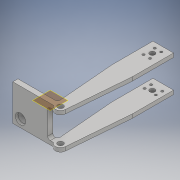
# Autodesk Inventor part: WheelIntakeMount3.0
Saved by Autodesk Inventor 2017 (Build 210142000, 142)
## iProperties
Created: 2017-12-06
Part Number: WheelIntakeMount3.0
Material: Generic
Document SubType Name: Modeling
Designer: User
Density: 1 g/cm^3
Appearance: Default
Author: User
Autodesk Inventor part; units mm, degrees
ref_plane "YZ Plane" through (0, 0, 0) normal (1, 0, 0) x (0, 1, 0)
ref_plane "XZ Plane" through (0, 0, 0) normal (0, 1, 0) x (-1, 0, 0)
ref_plane "XY Plane" through (0, 0, 0) normal (0, 0, 1) x (1, 0, 0)
sketch "Sketch1" plane through (0, 0, 0) normal (1, 0, 0) x (0, 1, 0)
  line L0 (0, 0) -> (127, 0)
  line L1 (127, 0) -> (127, -25.4)
  line L2 (127, -25.4) -> (0, -25.4)
  line L3 (0, -25.4) -> (0, 0)
  line L4 (0, -6.35) -> (0, -19.05)
  line L5 (0, -6.35) -> (76.2, 0)
  line L6 (0, -19.05) -> (76.2, -25.4)
  dimension "d0" = 127
  dimension "d1" = 25.4
  dimension "d18" = 12.7
  dimension "d19" = 6.35
  dimension "d20" = 50.8
  dimension "d21" = 50.8
  constraints: 14 end point, 4 point on line, 2 parallel, 1 horizontal, 1 perpendicular
  measures "d0" distance of L1.end L2.end
  measures "d1" distance of L0.end L1.end
  measures "d18" distance of L4.start L4.end
  measures "d19" distance from line of L2 L4.end
  measures "d20" distance from line of L1 L6.end
  measures "d21" distance from line of L5.end L1
ref_plane "Work Plane1" through (44.5262, 0, 0) normal (1, 0, 0) x (0, 0, -1)
sketch "Sketch2" plane through (44.5262, 0, 0) normal (1, 0, 0) x (0, 0, -1)
  line L0 (0, 127) -> (0, 0) projected
  line L1 (0, 0) -> (25.4, 0) projected
  line L2 (25.4, 0) -> (25.4, 127) projected
  line L3 (25.4, 127) -> (0, 127) projected
  line L4 (0, 0) -> (25.4, 0) projected
  circle A0 centre (12.7, 0) radius 6.35
  dimension "d5" = 25.4
  dimension "d6" = 12.7
  dimension "d7" = 12.7
  dimension "d8" = 0
  constraints: 1 centre point
  measures "d5" distance of L2.end L0.start
  measures "d6" diameter of A0
  measures "d7" distance from line of L2 A0.centre
  measures "d8" distance from line of A0.centre L1
extrude "Extrusion2" add sketch "Sketch2" against normal blind 44.5262 contours A0 L1 | L1 A0
ref_plane "Work Plane2" through (44.5262, 0, 0) normal (1, 0, 0) x (0, 0, -1)
extrude "Extrusion3" add sketch "Sketch1" along normal blind 44.5262 contours L0 L1 L2 L6 L3 L5
sketch "Sketch4" plane through (0, 0, 0) normal (-1, 0, 0) x (0, 0, 1)
  arc A0 (-19.05, 0) -> (-6.35, 0) centre (-12.7, 0) ccw projected
  line L0 (0, 76.2) -> (-6.35, 0) projected
  line L1 (0, 127) -> (0, 76.2) projected
  line L2 (-25.4, 127) -> (0, 127) projected
  line L3 (-25.4, 76.2) -> (-25.4, 127) projected
  line L4 (-19.05, 0) -> (-25.4, 76.2) projected
  point P0 (0, 0)
hole "Hole2" at (0, 0, -12.7) direction (1, 0, 0) diameter 6.858 end through all
sketch "Sketch5" plane through (0, 0, 0) normal (-1, 0, 0) x (0, 0, 1)
  circle A0 centre (-12.7, 0) radius 3.429 projected
  line L0 (0, 76.2) -> (-6.35, 0) projected
  line L1 (0, 127) -> (0, 76.2) projected
  line L2 (-25.4, 127) -> (0, 127) projected
  line L3 (-25.4, 76.2) -> (-25.4, 127) projected
  line L4 (-19.05, 0) -> (-25.4, 76.2) projected
  line L5 (-7.6835, 3.175) -> (43.1165, 3.175)
  line L6 (43.1165, 3.175) -> (43.1165, -3.175)
  line L7 (43.1165, -3.175) -> (-7.6835, -3.175)
  line L8 (-7.6835, -3.175) -> (-7.6835, 3.175)
  arc A1 (-19.05, 0) -> (-6.35, 0) centre (-12.7, 0) ccw projected
  point P0 (0, 0)
  dimension "d31" = 50.8
  dimension "d32" = 6.35
  dimension "d35" = 127
  dimension "d36" = 123.825
  dimension "d95" = 6.858
  dimension "d96" = 5.0165
  constraints: 8 end point, 2 parallel, 1 horizontal, 1 perpendicular
  measures "d31" distance of L6.end L7.end
  measures "d32" distance of L5.end L6.end
  measures "d35" distance from line of A0.centre L2
  measures "d36" distance between parallel lines of L2 L5
  measures "d95" diameter of A0
  measures "d96" distance from line of A0.centre L8
extrude "Extrusion4" add sketch "Sketch5" against normal blind 44.5262 contours L5 L6 L7 A1 L0 | L0 A1 L7 L8 L5
sketch "Sketch8" plane through (0, 76.2, -25.4) normal (0, 0, -1) x (-1, 0, 0)
  line L0 (0, 0) -> (0, 50.8) projected
  line L1 (0, 50.8) -> (-44.5262, 50.8) projected
  line L2 (-44.5262, 0) -> (-44.5262, 50.8) projected
  line L3 (0, 0) -> (-44.5262, 0) projected
  line L4 (0, -76.2) -> (0, 0) projected
  line L5 (0, 0) -> (-44.5262, 0) projected
  line L6 (-44.5262, -76.2) -> (-44.5262, 0) projected
  line L7 (0, 50.8) -> (-44.5262, 50.8) projected
  line L8 (-39.7637, 50.8) -> (-4.7625, 50.8)
  line L9 (-4.7625, 50.8) -> (-4.7625, -98.425)
  line L10 (-4.7625, -98.425) -> (-39.7637, -98.425)
  line L11 (-39.7637, -98.425) -> (-39.7637, 50.8)
  line L12 (0, -76.2) -> (-44.5262, -76.2) projected
  point P0 (0, -76.2)
  dimension "d41" = 44.5262
  dimension "d43" = 35.0012
  dimension "d44" = 4.7625
  dimension "d45" = 149.225
  constraints: 8 end point, 2 parallel, 1 horizontal, 1 perpendicular, 1 point on line
  measures "d41" distance of L0.end L1.end
  measures "d43" distance of L8.end L8.start
  measures "d44" distance between parallel lines of L0 L9
  measures "d45" distance between parallel lines of L10 L1
extrude "Extrusion5" cut sketch "Sketch8" against normal blind 25.4 contours L9 L12 L11 L3 | L3 L11 L1 L9 | L9 L10 L11 L12
fillet "Fillet1" radius 3.175 2 edges at (39.7637, 0, 0) (4.7625, 0, 0)
fillet "Fillet2" radius 3.175 2 edges at (2.3812, 3.175, -6.0854) (42.1449, 3.175, -6.0854)
sketch "Sketch9" plane through (0, 0, 0) normal (-1, 0, 0) x (0, 0, 1)
  line L0 (0, 76.2) -> (-5.7989, 6.6137) projected
  line L1 (0, 127) -> (0, 76.2) projected
  line L2 (-25.4, 127) -> (0, 127) projected
  line L3 (-25.4, 76.2) -> (-25.4, 127) projected
  line L4 (-19.05, 0) -> (-25.4, 76.2) projected
  circle A0 centre (-12.7, 0) radius 3.429 projected
  circle A1 centre (-12.7, 114.8637) radius 8
  line L5 (-19.6282, 118.8637) -> (-5.7718, 118.8637)
  line L6 (-5.7718, 118.8637) -> (-5.7718, 110.8637)
  line L7 (-5.7718, 110.8637) -> (-19.6282, 110.8637)
  line L8 (-19.6282, 110.8637) -> (-19.6282, 118.8637)
  arc A2 (-19.05, 0) -> (-7.2007, -3.175) centre (-12.7, 0) ccw projected
  line L9 (43.1165, -3.175) -> (-7.2007, -3.175) projected
  line L10 (43.1165, 3.175) -> (43.1165, -3.175) projected
  line L11 (-2.6348, 3.175) -> (43.1165, 3.175) projected
  arc A3 (-5.7989, 6.6137) -> (-2.6348, 3.175) centre (-2.6348, 6.35) ccw projected
  point P0 (0, 0)
  dimension "d50" = 16
  dimension "d51" = 25.4
  dimension "d52" = 12.7
  dimension "d53" = 8
  dimension "d54" = 4
  constraints: 8 end point, 2 parallel, 2 point on circle, 1 centre point, 1 horizontal, 1 perpendicular
  measures "d50" diameter of A1
  measures "d51" distance of L2.start L1.start
  measures "d52" distance from line of L1 A1.centre
  measures "d53" distance of L5.end L6.end
  measures "d54" distance from line of A1.centre L7
hole "Hole3" at (0, 118.8637, -19.6282) at (0, 110.8637, -19.6282) at (0, 118.8637, -5.7718) at (0, 110.8637, -5.7718) direction (1, 0, 0) diameter 2.9718 depth 25.4 tip angle 118
sketch "Sketch10" plane through (44.5262, 0, 0) normal (1, 0, 0) x (0, 0, -1)
  line L0 (19.05, 0) -> (25.4, 76.2) projected
  line L1 (25.4, 76.2) -> (25.4, 127) projected
  line L2 (25.4, 127) -> (0, 127) projected
  line L3 (0, 127) -> (0, 76.2) projected
  line L4 (0, 76.2) -> (5.7989, 6.6137) projected
  circle A0 centre (12.7, 0) radius 3.429 projected
  circle A1 centre (12.7, 113.546) radius 8
  line L5 (16.7, 106.6178) -> (8.7, 106.6178)
  line L6 (8.7, 106.6178) -> (8.7, 120.4742)
  line L7 (8.7, 120.4742) -> (16.7, 120.4742)
  line L8 (16.7, 120.4742) -> (16.7, 106.6178)
  arc A2 (7.2007, -3.175) -> (19.05, 0) centre (12.7, 0) ccw projected
  arc A3 (2.6348, 3.175) -> (5.7989, 6.6137) centre (2.6348, 6.35) ccw projected
  line L9 (2.6348, 3.175) -> (-43.1165, 3.175) projected
  line L10 (-43.1165, 3.175) -> (-43.1165, -3.175) projected
  line L11 (-43.1165, -3.175) -> (7.2007, -3.175) projected
  point P0 (0, 0)
  dimension "d62" = 16
  dimension "d63" = 25.4
  dimension "d64" = 12.7
  dimension "d65" = 8
  dimension "d66" = 4
  constraints: 8 end point, 2 parallel, 2 point on circle, 1 centre point, 1 horizontal, 1 perpendicular
  measures "d62" diameter of A1
  measures "d63" distance of L1.end L2.end
  measures "d64" distance from line of L3 A1.centre
  measures "d65" distance of L5.start L5.end
  measures "d66" distance from line of L6 A1.centre
hole "Hole4" at (44.5262, 106.6178, -16.7) at (44.5262, 106.6178, -8.7) at (44.5262, 120.4742, -8.7) at (44.5262, 120.4742, -16.7) direction (-1, 0, 0) diameter 2.9718 depth 25.4 tip angle 118
sketch "Sketch11" plane through (0, -3.175, -7.2007) normal (0, -1, 0) x (1, 0, 0)
  line L0 (4.7625, 0) -> (4.7625, 4.0257) projected
  arc A0 (7.9375, 7.2007) -> (4.7625, 4.0257) centre (7.9375, 4.0257) ccw projected
  line L1 (7.9375, 7.2007) -> (36.5887, 7.2007) projected
  arc A1 (39.7637, 4.0257) -> (36.5887, 7.2007) centre (36.5887, 4.0257) ccw projected
  line L2 (39.7637, 4.0257) -> (39.7637, 0) projected
  line L3 (44.5262, 50.3172) -> (44.5262, 0) projected
  line L4 (0, 50.3172) -> (44.5262, 50.3172) projected
  line L5 (0, 50.3172) -> (0, 0) projected
  line L6 (44.5262, 0) -> (39.7637, 0) projected
  line L7 (4.7625, 0) -> (0, 0) projected
  point P0 (0, 7.2007)
  point P1 (9.525, 40.7922)
  dimension "d74" = 9.525
  dimension "d75" = 44.5262
  dimension "d97" = 9.525
  measures "d74" distance from line of L4 point (9.525, 40.792)
  measures "d75" distance of L4.start L3.start
  measures "d97" distance from line of L5 point (9.525, 40.792)
hole "Hole5" at (9.525, -3.175, 33.5915) direction (0, 1, 0) diameter 12.7 depth 3.175 tip angle 118
sketch "Sketch12" plane through (44.5262, 0, 0) normal (1, 0, 0) x (0, 0, -1)
  circle A0 centre (8.7, 120.4742) radius 1.4859 projected
  circle A1 centre (16.7, 106.6178) radius 1.4859 projected
  circle A2 centre (8.7, 106.6178) radius 1.4859 projected
  circle A3 centre (16.7, 120.4742) radius 1.4859 projected
  line L0 (19.05, 0) -> (25.4, 76.2) projected
  line L1 (25.4, 76.2) -> (25.4, 127) projected
  line L2 (25.4, 127) -> (0, 127) projected
  line L3 (0, 127) -> (0, 76.2) projected
  line L4 (0, 76.2) -> (5.7989, 6.6137) projected
  circle A4 centre (12.7, 0) radius 3.429 projected
  arc A5 (7.2007, -3.175) -> (19.05, 0) centre (12.7, 0) ccw projected
  arc A6 (2.6348, 3.175) -> (5.7989, 6.6137) centre (2.6348, 6.35) ccw projected
  line L5 (2.6348, 3.175) -> (-43.1165, 3.175) projected
  line L6 (-43.1165, 3.175) -> (-43.1165, -3.175) projected
  line L7 (-43.1165, -3.175) -> (7.2007, -3.175) projected
  point P0 (0, 0)
  point P1 (12.7, 113.546)
  dimension "d84" = 25.4
  dimension "d85" = 12.7
  dimension "d86" = 13.8564
  dimension "d87" = 6.9282
  measures "d84" distance of L1.end L2.end
  measures "d85" distance from line of L3 point (12.7, 113.546)
  measures "d86" distance of A2.centre A0.centre
  measures "d87" vertical distance of A2.centre point (12.7, 113.546)
hole "Hole6" at (44.5262, 113.546, -12.7) direction (-1, 0, 0) diameter 6.35 end through all
equation "\"d19\" = -0.5 * d18 + 0.5 * d1"
equation "\"d21\" = d20"
equation "\"d7\" = 0.5 * d5"
equation "\"d36\" = d35 - 0.5 * d32"
equation "\"d44\" = -0.5 * d43 + 0.5 * d41"
equation "\"d52\" = 0.5 * d51"
equation "\"d54\" = 0.5 * d53"
equation "\"d64\" = 0.5 * d63"
equation "\"d66\" = 0.5 * d65"
equation "\"d87\" = 0.5 * d86"
body "Solid1"
